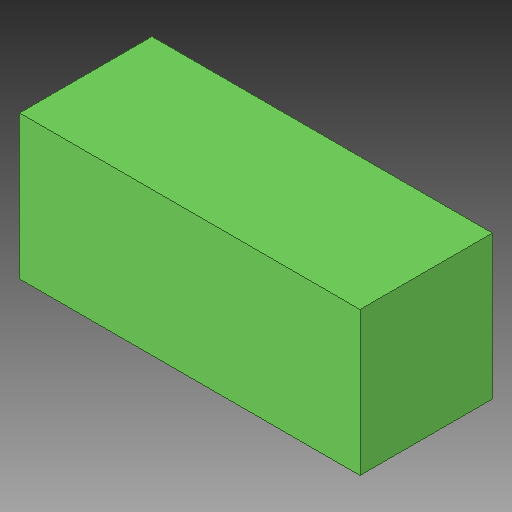
# Autodesk Inventor part: Multistar-6S-16Ah
Saved by Autodesk Inventor 2019.2 (Build 232265000, 265)
## iProperties
Created: 2018-09-23
Part Number: Multistar-6S-16Ah
Material: Generic
Document SubType Name: Modeling
Designer: eroldan
Density: 1 g/cm^3
Appearance: Default
Author: eroldan
Autodesk Inventor part; units mm, degrees
ref_plane "YZ Plane" through (0, 0, 0) normal (1, 0, 0) x (0, 1, 0)
ref_plane "XZ Plane" through (0, 0, 0) normal (0, 1, 0) x (-1, 0, 0)
ref_plane "XY Plane" through (0, 0, 0) normal (0, 0, 1) x (1, 0, 0)
sketch "Sketch1" plane through (0, 0, 0) normal (0, 0, 1) x (1, 0, 0)
  line L0 (-90, -38) -> (90, -38)
  line L1 (90, -38) -> (90, 38)
  line L2 (90, 38) -> (-90, 38)
  line L3 (-90, 38) -> (-90, -38)
  line L4 (-90, -38) -> (90, 38) construction
  line L5 (90, -38) -> (-90, 38) construction
  point P0 (0, 0)
  dimension "d0" = 180
  dimension "d1" = 76
  constraints: 12 end point, 2 midpoint, 2 parallel, 1 horizontal, 1 perpendicular
  measures "d0" distance of L2.end L1.end
  measures "d1" distance of L1.end L0.end
extrude "Extrusion1" add sketch "Sketch1" along normal mid plane 70
fillet "Fillet1" [suppressed]
body "Solid1"
